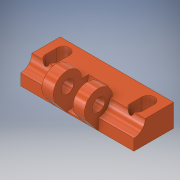
# Autodesk Inventor part: Piston Wall Guide Wide
Saved by Autodesk Inventor 2018 (Build 220112000, 112)
## iProperties
Created: 2017-09-27
Part Number: Piston Wall Guide Wide
Material: ABS Plastic
Document SubType Name: Modeling
Designer: Gabriel Smolnycki
Density: 1.06 g/cm^3
Appearance: Smooth - Light Orange
Author: Gabriel Smolnycki
Autodesk Inventor part; units mm, degrees
ref_plane "YZ Plane" through (0, 0, 0) normal (1, 0, 0) x (0, 1, 0)
ref_plane "XZ Plane" through (0, 0, 0) normal (0, 1, 0) x (-1, 0, 0)
ref_plane "XY Plane" through (0, 0, 0) normal (0, 0, 1) x (1, 0, 0)
sketch "Sketch1" plane through (0, 0, 0) normal (0, 1, 0) x (-1, 0, 0)
  line L0 (7.5, 7) -> (-7.5, 7)
  line L1 (-7.5, 7) -> (-7.5, -7)
  line L2 (-7.5, -7) -> (7.5, -7)
  line L3 (7.5, -7) -> (7.5, 7)
  line L4 (7.5, 7) -> (-7.5, -7) construction
  line L5 (-7.5, 7) -> (7.5, -7) construction
  point P0 (0, 0)
  dimension "d0" = 15
  dimension "d1" = 14
  constraints: 12 end point, 2 midpoint, 2 parallel, 1 horizontal, 1 perpendicular
  measures "d0" distance of L2.end L1.end
  measures "d1" distance of L1.end L0.end
extrude "Extrusion1" add sketch "Sketch1" along normal blind 8
sketch "Sketch2" plane through (7.5, 0, 7) normal (1, 0, 0) x (0, 0, -1)
  line L0 (0, 8) -> (14, 8) projected
  line L1 (0, 0) -> (0, 8) projected
  arc A0 (5, 8) -> (-3.9031, 4.875) centre (0, 8) ccw
  line L2 (0, 0) -> (-3.9031, 4.875)
  point P0 (7, 0)
  dimension "d4" = 10
  constraints: 2 end point, 2 point on circle, 1 centre point, 1 coincident, 1 point on line
  measures "d4" diameter of A0
extrude "Extrusion2" add sketch "Sketch2" against normal blind 4
mirror "Mirror1" about plane through (0, 0, 0) normal (1, 0, 0) of "Extrusion2"
sketch "Sketch3" plane through (3.5, 0, 7) normal (-1, 0, 0) x (0, 0, 1)
  arc A0 (3.9031, 4.875) -> (-5, 8) centre (0, 8) ccw projected
  circle A1 centre (0, 8) radius 7.5
  point P0 (-7, 0)
  dimension "d7" = 15
  constraints: 1 centre point, 1 coincident
  measures "d7" diameter of A1
extrude "Extrusion3" cut sketch "Sketch3" along normal up to surface (7 mm away)
sketch "Sketch4" plane through (7.5, 0, -7) normal (1, 0, 0) x (0, 0, -1)
  line L0 (0, 0) -> (0, 8) projected
  line L1 (0, 0) -> (-14, 0)
  line L2 (-14, 0) -> (-14, 4)
  line L3 (-10, 8) -> (0, 8)
  line L4 (0, 8) -> (0, 0)
  arc A0 (-14, 4) -> (-10, 8) centre (-14, 8) ccw
  point P0 (-7, 0)
  dimension "d12" = 8
  dimension "d13" = 8
  dimension "d14" = 14
  constraints: 8 end point, 2 parallel, 2 point on circle, 1 centre point, 1 horizontal, 1 horizontal alignment, 1 perpendicular, 1 vertical alignment
  measures "d12" diameter of A0
  measures "d13" distance between parallel lines of L1 L3
  measures "d14" distance between parallel lines of L2 L0
extrude "Extrusion4" add sketch "Sketch4" along normal blind 12.5
sketch "Sketch5" plane through (0, 8, 0) normal (0, 1, 0) x (1, 0, 0)
  line L0 (15, -1) -> (15, 3) construction
  line L1 (17.25, -1) -> (17.25, 3)
  line L2 (12.75, 3) -> (12.75, -1)
  arc A0 (12.75, -1) -> (17.25, -1) centre (15, -1) ccw
  arc A1 (17.25, 3) -> (12.75, 3) centre (15, 3) ccw
  line L3 (-7.5, 7) -> (20, 7) projected
  point P0 (0, 0)
  point P1 (15, 1)
  dimension "d17" = 4
  dimension "d18" = 4.5
  dimension "d19" = 15
  dimension "d20" = 6
  constraints: 8 end point, 4 point on circle, 4 tangent, 2 centre point, 1 midpoint, 1 parallel, 1 vertical
  measures "d17" distance of L0.start L0.end
  measures "d18" diameter of A1
  measures "d19" horizontal distance of point (15, 1) point (0, 0)
  measures "d20" distance from line of L3 point (15, 1)
extrude "Extrusion5" cut sketch "Sketch5" against normal through all
mirror "Mirror2" about plane through (0, 0, 0) normal (1, 0, 0) of "Extrusion5", "Extrusion4"
sketch "Sketch6" plane through (7.5, 0, 7) normal (1, 0, 0) x (0, 0, -1)
  arc A0 (5, 8) -> (-3.9031, 4.875) centre (0, 8) ccw projected
  point P0 (7, 0)
  constraints: 1 coincident
hole "Hole1" at (7.5, 8, 7) direction (-1, 0, 0) diameter 4.5 end through all
body "Solid1"
